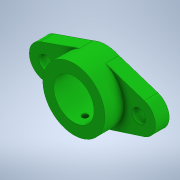
# Autodesk Inventor part: Chumacera
Saved by Autodesk Inventor 2020 (Build 240168000, 168)
## iProperties
Created: 2019-10-03
Part Number: Chumacera
Material: Genérico
Document SubType Name: Modeling
Designer: Everardo
Density: 1 g/cm^3
Appearance: Verde oscuro
Author: Everardo
Autodesk Inventor part; units mm, degrees
ref_plane "YZ Plane" through (0, 0, 0) normal (1, 0, 0) x (0, 1, 0)
ref_plane "XZ Plane" through (0, 0, 0) normal (0, 1, 0) x (-1, 0, 0)
ref_plane "XY Plane" through (0, 0, 0) normal (0, 0, 1) x (1, 0, 0)
sketch "Boceto1" plane through (0, 0, 0) normal (0, 0, 1) x (1, 0, 0)
  circle A0 centre (-27.7266, -0.9426) radius 7
  circle A1 centre (-20, 3.239) radius 0.1677
  circle A2 centre (68.2698, -0.1077) radius 7
  arc A3 (73.4655, -16.2943) -> (73.5445, 16.0533) centre (68.2698, -0.1077) ccw
  circle A4 centre (20.2642, 0) radius 32
  line L0 (-33.3043, 15.1163) -> (6.9422, 29.0951)
  line L1 (73.5445, 16.0533) -> (33.5861, 29.0951)
  line L2 (-33.0105, -17.1059) -> (6.9422, -29.0951)
  line L3 (73.4655, -16.2943) -> (33.5861, -29.0951)
  arc A5 (-33.3043, 15.1163) -> (-32.6128, -17.2252) centre (-27.7266, -0.9426) ccw
  point P0 (0, 0)
  dimension "d0" = 14
  dimension "d2" = 14
  dimension "d3" = 96
  dimension "d5" = 34
  dimension "d6" = 64
  dimension "d7" = 48
  constraints: 8 end point, 8 point on circle, 6 centre point, 4 tangent, 2 coincident, 1 point on line
  measures "d0" diameter of A0
  measures "d2" diameter of A2
  measures "d3" distance of A2.centre A0.centre
  measures "d5" diameter of A3
  measures "d6" diameter of A4
  measures "d7" distance of A4.centre A0.centre
extrude "Extrusión1" add sketch "Boceto1" along normal blind 14 contours L3 A4 L1 A3 | L2 A5 L0 A4
extrude "Extrusión3" add sketch "Boceto1" along normal blind 33 contours A4
sketch "Boceto4" plane through (20.2642, 0, 33) normal (0, 0, 1) x (1, 0, 0)
  circle A0 centre (0, 0) radius 20.64
  point P0 (-20.2642, 0)
  dimension "d21" = 41.28
  constraints: 1 centre point
  measures "d21" diameter of A0
extrude "Extrusión4" cut sketch "Boceto4" against normal through all
sketch "Boceto5" plane through (0, 0, 0) normal (0, 1, 0) x (-1, 0, 0)
  line L0 (-40.9042, 33) -> (0.3758, 33) projected
  line L1 (0.3758, 0) -> (-40.9042, 0) projected
  line L2 (-40.9042, 33) -> (0.3758, 33) projected
  line L3 (0.3758, 0) -> (-40.9042, 0) projected
  line L4 (-40.9042, 33) -> (0.3758, 33) projected
  line L5 (0.3758, 0) -> (-40.9042, 0) projected
  line L6 (-40.9042, 33) -> (0.3758, 33) projected
  line L7 (-20.3915, 34.6516) -> (-20.3915, 21.6516)
  line L8 (11.7358, 33) -> (-52.2642, 33) projected
  line L9 (-20.3915, 34.6516) -> (-7.3915, 34.6516) construction
  circle A0 centre (-20.3915, 21.6516) radius 3
  point P0 (0, 0)
  point P1 (-20.2642, 0)
  dimension "d24" = 13
  dimension "d25" = 90
  dimension "d26" = 6
  constraints: 4 end point, 1 centre point, 1 coincident, 1 horizontal, 1 perpendicular, 1 vertical, 1 other
  measures "d24" distance of L7.start L7.end
  measures "d25" angle of L7 L9
  measures "d26" diameter of A0
extrude "Extrusión5" cut sketch "Boceto5" against normal blind 33
